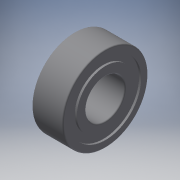
# Autodesk Inventor part: BR115ZZ
Saved by Autodesk Inventor 2018.1 (Build 221171000, 171)
## iProperties
Category: PARTsolutions
Company: MISUMI
Created: 2018-12-11
Part Number: BR115ZZ
Material: Generic
Catalog Web Link: www.cadenas.de
Description: B6 _ _ ZZ, B6 _ _ AZZ, SB6 _ _ ZZ, SB6 _ _ AZZ, BR _ _ ZZ, SBR _ _ ZZ-Small Ball Bearings - Double Shield Type
Vendor: MISUMI
Document SubType Name: Modeling
Designer: psadmin
Manufacturer: MISUMI
Mass: 0.288595 g
Surface Area: 3.73038 cm^2
Volume: 0.288595 cm^3
Density: 1 g/cm^3
Appearance: PSOLRGB-175-175-175
PSOL_IDENT_0: {$CADENAS_DATA\23d-libs\misumi\metric\12_bearing_holders\sb685zz.prj},221 {VTYP=3D},{NB=BR115ZZ},{LI
PSOL_IDENT_1: NA=BR115ZZ},{NN=B6 _ _ ZZ, B6 _ _ AZZ, SB6 _ _ ZZ, SB6 _ _ AZZ, BR _ _ ZZ, SBR _ _ ZZ},{DATE=30.03.2
PSOL_IDENT_2: 018 01:49:31},{GEOMDATE=23.07.2013 00:00:00},{VERSION=},{LINEID=440},{WBVAR=MAT},{WBNUMERIC=}  {NB=B
PSOL_IDENT_3: R115ZZ},{LINA=BR115ZZ},{KT=DUMMY},{PN=BR115ZZ},{MAT=},{BN=115ZZ},{DD=5.0},{A=3.4688},{BB=0.905},{C=1
PSOL_IDENT_4: .190},{D=11},{B=4.0},{RR=0.15},{CR=716},{COR=282},{CRS=716},{CRSS=609},{CORS=282},{CORSS=226},{DS=6.
PSOL_IDENT_5: 81},{DDHH=9.90},{R=0.15},{MASS=0.62},{X=1},{BN2=B115ZZ}
NN: B6 _ _ ZZ, B6 _ _ AZZ, SB6 _ _ ZZ, SB6 _ _ AZZ, BR _ _ ZZ, SBR _ _ ZZ
NT: Small Ball Bearings - Double Shield Type
NB: BR115ZZ
NBSYN: $PN.
LINA: BR115ZZ
PN: BR115ZZ
MAT: 52100 Bearing Steel
BN: 115ZZ
DD: 5
D: 11
B: 4
RR: 0.15
CR: 716
COR: 282
DS: 6.81
DDHH: 9.9
R: 0.15
MASS: 0.62
X: 1
SUPPLIER: MISUMI
ARTICLENO: BR115ZZ
BOMINFO: BR115ZZ
CREATOR: CADENAS GmbH
Title: BR115ZZ
Author: Cadenas PARTsolutions
Comments: Small Ball Bearings - Double Shield Type
Autodesk Inventor part; units mm, degrees
ref_plane "YZ Plane" through (0, 0, 0) normal (1, 0, 0) x (0, 1, 0)
ref_plane "XZ Plane" through (0, 0, 0) normal (0, 1, 0) x (-1, 0, 0)
ref_plane "XY Plane" through (0, 0, 0) normal (0, 0, 1) x (1, 0, 0)
sketch "Sketch_1" plane through (0, 0, 0) normal (0, 0, 1) x (1, 0, 0)
  line L0 (3.85, 0) -> (0.15, 0)
  arc A0 (0, 2.65) -> (0.15, 2.5) centre (0.15, 2.65) ccw
  line L1 (0.15, 2.5) -> (3.85, 2.5)
  arc A1 (3.85, 2.5) -> (4, 2.65) centre (3.85, 2.65) ccw
  line L2 (4, 2.65) -> (4, 3.69)
  line L3 (4, 3.69) -> (3.7344, 3.69)
  line L4 (3.7344, 3.69) -> (3.7344, 4.595)
  line L5 (3.7344, 4.595) -> (4, 4.595)
  line L6 (4, 4.595) -> (4, 5.35)
  arc A2 (4, 5.35) -> (3.85, 5.5) centre (3.85, 5.35) ccw
  line L7 (3.85, 5.5) -> (0.15, 5.5)
  arc A3 (0.15, 5.5) -> (0, 5.35) centre (0.15, 5.35) ccw
  line L8 (0, 5.35) -> (0, 4.595)
  line L9 (0, 4.595) -> (0.2656, 4.595)
  line L10 (0.2656, 4.595) -> (0.2656, 3.69)
  line L11 (0.2656, 3.69) -> (0, 3.69)
  line L12 (0, 3.69) -> (0, 2.65)
  constraints: 26 end point, 8 point on circle, 4 centre point
revolve "Revolution1" add sketch "Sketch_1" angle 360 about axis through (3.85, 0, 0) along (1, 0, 0)
ref_plane "to_housing_XY" through (0, 0, 0) normal (1, 0, 0) x (0, 0, -1)
ref_plane "to_housing_YZ" through (0, 0, 0) normal (0, 0, -1) x (0, 1, 0)
ref_plane "to_housing_ZX" through (0, 0, 0) normal (0, 1, 0) x (1, 0, 0)
ref_plane "to_housing_center_XY" through (2, 0, 0) normal (1, 0, 0) x (0, 0, -1)
ref_plane "to_housing_center_YZ" through (2, 0, 0) normal (0, 0, -1) x (0, 1, 0)
ref_plane "to_housing_center_ZX" through (2, 0, 0) normal (0, 1, 0) x (1, 0, 0)
body "Solid1"
